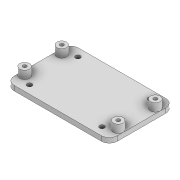
# Autodesk Inventor part: RaspberryMount
Saved by Autodesk Inventor 2022 (Build 260153000, 153)
## iProperties
Created: 2022-10-26
Part Number: RaspberryMount
Material: Generic
Document SubType Name: Modeling
Designer: MVeszpremi
Density: 1 g/cm^3
Appearance: Default
Author: MVeszpremi
Autodesk Inventor part; units mm, degrees
ref_plane "YZ Plane" through (0, 0, 0) normal (1, 0, 0) x (0, 1, 0)
ref_plane "XZ Plane" through (0, 0, 0) normal (0, 1, 0) x (-1, 0, 0)
ref_plane "XY Plane" through (0, 0, 0) normal (0, 0, 1) x (1, 0, 0)
sketch "Sketch1" plane through (0, 0, 0) normal (0, 1, 0) x (-1, 0, 0)
  line L0 (0, 0) -> (58, 0)
  line L1 (58, 0) -> (58, -23)
  line L2 (58, -23) -> (0, -23)
  line L3 (0, -23) -> (0, 0)
  line L4 (6.5, 3.5) -> (51.5, 3.5)
  line L5 (51.5, 3.5) -> (51.5, -26.5)
  line L6 (51.5, -26.5) -> (6.5, -26.5)
  line L7 (6.5, -26.5) -> (6.5, 3.5)
  circle A0 centre (51.5, 3.5) radius 1.5
  circle A1 centre (51.5, -26.5) radius 1.5
  circle A2 centre (6.5, -26.5) radius 1.5
  circle A3 centre (6.5, 3.5) radius 1.5
  line L8 (-3, 8.5) -> (61, 8.5)
  line L9 (61, 8.5) -> (61, -31.5)
  line L10 (61, -31.5) -> (-3, -31.5)
  line L11 (-3, -31.5) -> (-3, 8.5)
  circle A4 centre (58, 0) radius 1.15
  circle A5 centre (58, -23) radius 1.15
  circle A6 centre (0, 0) radius 1.15
  circle A7 centre (0, -23) radius 1.15
  circle A8 centre (58, 0) radius 3
  circle A9 centre (58, -23) radius 3
  circle A10 centre (0, 0) radius 3
  circle A11 centre (0, -23) radius 3
  dimension "d0" = 23
  dimension "d1" = 58
  dimension "d2" = 45
  dimension "d3" = 30
  dimension "d4" = 3.5
  dimension "d6" = 3
  dimension "d7" = 3
  dimension "d8" = 3
  dimension "d9" = 3
  dimension "d10" = 9.5
  dimension "d11" = 5
  dimension "d12" = 5
  dimension "d13" = 9.5
  dimension "d14" = 2.3
  dimension "d15" = 2.3
  dimension "d16" = 2.3
  dimension "d17" = 2.3
  dimension "d18" = 6
  dimension "d19" = 6
  dimension "d20" = 6
  dimension "d21" = 6
  dimension "d28" = 6.5
  constraints: 24 end point, 12 centre point, 12 coincident, 6 parallel, 3 horizontal, 3 perpendicular
  measures "d0" distance of L0.end L1.end
  measures "d1" distance of L1.end L2.end
  measures "d2" distance of L4.start L4.end
  measures "d3" distance of L4.end L5.end
  measures "d4" distance between parallel lines of L4 L0
  measures "d6" diameter of A0
  measures "d7" diameter of A1
  measures "d8" diameter of A2
  measures "d9" diameter of A3
  measures "d10" distance between parallel lines of L5 L9
  measures "d11" distance between parallel lines of L4 L8
  measures "d12" distance between parallel lines of L10 L6
  measures "d13" distance between parallel lines of L11 L7
  measures "d14" diameter of A4
  measures "d15" diameter of A5
  measures "d16" diameter of A6
  measures "d17" diameter of A7
  measures "d18" diameter of A10
  measures "d19" diameter of A11
  measures "d20" diameter of A8
  measures "d21" diameter of A9
  measures "d28" distance between parallel lines of L7 L3
extrude "Extrusion1" add sketch "Sketch1" along normal blind 3 contours A6 L3 A10 L0 | L0 A10 L3 A6 | A10 L11 L8 L9 A8 L0 L5 A0 L4 A3 L7 | L0 L7 L2 A11 L3 A10 | L3 A11 L11 A10 | L7 A3 L4 A0 L5 L0 | L0 L5 L2 L7 | A11 L2 A7 L3 | L3 A7 L2 A11 | L0 A8 L1 A9 L2 L5 | L7 A2 L6 A1 L5 L2 A9 L9 L10 L11 A11 | L2 L5 A1 L6 A2 L7 | A8 L1 A4 L0 | L0 A4 L1 A8 | L9 A9 L1 A8 | A9 L1 A5 L2 | L2 A5 L1 A9
extrude "Extrusion2" add sketch "Sketch1" along normal blind 8 contours A6 L3 A10 L0 | L0 A10 L3 A6 | A11 L2 A7 L3 | L3 A7 L2 A11 | A8 L1 A4 L0 | L0 A4 L1 A8 | A9 L1 A5 L2 | L2 A5 L1 A9
fillet "Fillet1" radius 5 4 edges at (-61, 1.5, 8.5) (3, 1.5, 8.5) (3, 1.5, -31.5) (-61, 1.5, -31.5)
body "Solid1"
